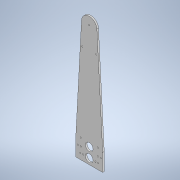
# Autodesk Inventor part: 関節3_側板2
Saved by Autodesk Inventor 2021 (Build 250183000, 183)
## iProperties
Created: 2022-01-31
Part Number: 関節3_側板2
Material: 一般
Document SubType Name: Modeling
Designer: hirohumi
Density: 1 g/cm^3
Appearance: 既定
Author: hirohumi
Autodesk Inventor part; units mm, degrees
ref_plane "YZ Plane" through (0, 0, 0) normal (1, 0, 0) x (0, 1, 0)
ref_plane "XZ Plane" through (0, 0, 0) normal (0, 1, 0) x (-1, 0, 0)
ref_plane "XY Plane" through (0, 0, 0) normal (0, 0, 1) x (1, 0, 0)
sketch "スケッチ1" plane through (0, 0, 0) normal (0, 0, 1) x (1, 0, 0)
  circle A0 centre (0, 0) radius 50 construction
  circle A1 centre (0, 25) radius 11.9375 construction
  circle A2 centre (0, 300) radius 5 construction
  circle A3 centre (0, 300) radius 47.7465 construction
  line L0 (47.4805, 294.9672) -> (13.1081, -29.3118) construction
  line L1 (-47.4611, 294.7873) -> (-11.8661, -29.3033) construction
  circle A4 centre (0, 25) radius 19.25 construction
  line L2 (-12.0776, 316.763) -> (11.6547, 316.763) construction
  line L3 (-22.6185, -92.0395) -> (22.1946, -92.0395) construction
  circle A5 centre (0, 300) radius 1.75
  arc A6 (35, 30) -> (34.9923, 30.2769) centre (30, 30) ccw
  arc A7 (-34.9923, 30.2769) -> (-35, 30) centre (-30, 30) ccw
  arc A8 (19.9693, 301.1077) -> (-19.9693, 301.1077) centre (0, 300) ccw
  line L4 (-19.9693, 301.1077) -> (-34.9923, 30.2769)
  line L5 (19.9693, 301.1077) -> (34.9923, 30.2769)
  line L6 (-35, 30) -> (-35, -15)
  line L7 (35, -15) -> (35, 30)
  circle A9 centre (-9.1924, 34.1924) radius 1.6 construction
  circle A10 centre (9.1924, 34.1924) radius 1.6 construction
  line L8 (9.1924, 34.1924) -> (-9.1924, 34.1924) construction
  line L9 (-9.1924, 34.1924) -> (-9.1924, 15.8076) construction
  line L10 (-9.1924, 15.8076) -> (9.1924, 15.8076) construction
  line L11 (9.1924, 15.8076) -> (9.1924, 34.1924) construction
  line L12 (9.1924, 34.1924) -> (-9.1924, 15.8076) construction
  line L13 (-9.1924, 34.1924) -> (9.1924, 15.8076) construction
  circle A11 centre (0, 25) radius 13 construction
  circle A12 centre (-9.1924, 15.8076) radius 1.6 construction
  circle A13 centre (9.1924, 15.8076) radius 1.6 construction
  circle A14 centre (0, 25) radius 10.05
  circle A15 centre (0, 0) radius 4 construction
  circle A16 centre (0, 0) radius 10
  line L14 (22.5, 35) -> (-22.5, 35) construction
  line L15 (-22.5, 35) -> (-22.5, 15) construction
  line L16 (-22.5, 15) -> (22.5, 15) construction
  line L17 (22.5, 15) -> (22.5, 35) construction
  line L18 (22.5, 35) -> (-22.5, 15) construction
  line L19 (-22.5, 35) -> (22.5, 15) construction
  circle A17 centre (-22.5, 35) radius 1.6
  circle A18 centre (-22.5, 15) radius 1.6
  circle A19 centre (22.5, 35) radius 1.6
  circle A20 centre (22.5, 15) radius 1.6
  circle A21 centre (0, 0) radius 16.215 construction
  circle A22 centre (0, 0) radius 23.0125 construction
  circle A23 centre (-23.0125, 0) radius 1.6
  circle A24 centre (-16.215, 0) radius 1.6
  circle A25 centre (16.215, 0) radius 1.6
  circle A26 centre (23.0125, 0) radius 1.6
  line L20 (-35, -15) -> (35, -15)
  line L21 (30, 30) -> (-30, 30) construction
  line L22 (-30, 30) -> (-30, -30) construction
  line L23 (-30, -30) -> (30, -30) construction
  line L24 (30, -30) -> (30, 30) construction
  line L25 (30, 30) -> (-30, -30) construction
  line L26 (-30, 30) -> (30, -30) construction
  circle A27 centre (-30, 15) radius 1.6
  circle A28 centre (30, 15) radius 1.6
  circle A29 centre (0, 300) radius 60 construction
  circle A30 centre (-18, 242.7636) radius 1.6
  circle A31 centre (18, 242.7636) radius 1.6
  dimension "d38" = 26
  dimension "d1" = 100
  dimension "d3" = 23.875
  dimension "d8" = 10
  dimension "d9" = 300
  dimension "d10" = 95.493
  dimension "d11" = 38.5
  dimension "d25" = 3.5
  dimension "d26" = 5
  dimension "d28" = 20
  dimension "d29" = 5
  dimension "d35" = 25
  dimension "d36" = 3.2
  dimension "d37" = 3.2
  dimension "d39" = 3.2
  dimension "d40" = 3.2
  dimension "d41" = 20.1
  dimension "d42" = 8
  dimension "d43" = 20
  dimension "d44" = 45
  dimension "d45" = 20
  dimension "d46" = 3.2
  dimension "d47" = 3.2
  dimension "d48" = 3.2
  dimension "d49" = 3.2
  dimension "d52" = 32.43
  dimension "d53" = 46.025
  dimension "d54" = 3.2
  dimension "d55" = 3.2
  dimension "d56" = 3.2
  dimension "d57" = 3.2
  dimension "d58" = 15
  dimension "d59" = 60
  dimension "d60" = 60
  dimension "d61" = 3.2
  dimension "d62" = 3.2
  dimension "d63" = 15
  dimension "d64" = 15
  dimension "d65" = 120
  dimension "d66" = 3.2
  dimension "d67" = 3.2
  dimension "d68" = 36
  constraints: 54 end point, 31 centre point, 25 coincident, 14 point on circle, 8 tangent, 7 parallel, 6 horizontal, 6 midpoint, 5 horizontal alignment, 4 perpendicular, 3 point on line, 2 vertical alignment, 1 vertical, 3 other
  measures "d1" diameter of A0
  measures "d3" diameter of A1
  measures "d8" diameter of A2
  measures "d9" distance of point (0, 0) A2.centre
  measures "d10" diameter of A3
  measures "d11" diameter of A4
  measures "d25" diameter of A5
  measures "d26" radius of A6
  measures "d28" radius of A8
  measures "d29" radius of A7
  measures "d35" distance of point (0, 0) A1.centre
  measures "d36" diameter of A9
  measures "d37" diameter of A10
  measures "d39" diameter of A12
  measures "d40" diameter of A13
  measures "d41" diameter of A14
  measures "d42" diameter of A15
  measures "d43" diameter of A16
  measures "d44" distance of L16.end L15.end
  measures "d45" distance of L15.end L14.end
  measures "d46" diameter of A17
  measures "d47" diameter of A18
  measures "d48" diameter of A19
  measures "d49" diameter of A20
  measures "d52" diameter of A21
  measures "d53" diameter of A22
  measures "d54" diameter of A23
  measures "d55" diameter of A24
  measures "d56" diameter of A25
  measures "d57" diameter of A26
  measures "d58" distance from line of L20 point (0, 0)
  measures "d59" distance of L23.end L22.end
  measures "d60" distance of L22.end L21.end
  measures "d61" diameter of A27
  measures "d62" diameter of A28
  measures "d63" distance of A28.centre A6.centre
  measures "d64" distance of A27.centre A7.centre
  measures "d65" diameter of A29
  measures "d66" diameter of A30
  measures "d67" diameter of A31
  measures "d68" distance of A31.centre A30.centre
extrude "押し出し2" add sketch "スケッチ1" along normal blind 4
